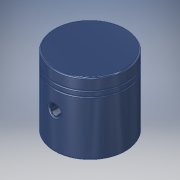
# Autodesk Inventor part: Se-Elmer-Radical-Engine:Piston
Saved by Autodesk Inventor 2017 (Build 210142000, 142)
## iProperties
Created: 2020-01-12
Material: Stainless Steel
Document SubType Name: Modeling
Designer: Admin
Density: 8 g/cm^3
Appearance: Flaked Satin - Blue
Mass: 15.0776 g
Surface Area: 16.4031 cm^2
Volume: 1.88469 cm^3
Author: Admin
Autodesk Inventor part; units mm, degrees
ref_plane "YZ Plane" through (0, 0, 0) normal (1, 0, 0) x (0, 1, 0)
sketch "Sketch1" plane through (0, 0, 0) normal (0, 1, 0) x (-1, 0, 0)
  circle A0 centre (0, 0) radius 7.9375
  dimension "d0" = 15.875
  constraints: 1 centre point, 1 coincident
  measures "d0" diameter of A0
extrude "Extrusion1" add sketch "Sketch1" along normal mid plane 15.875
sketch "Sketch2" plane through (0, -7.9375, 0) normal (0, -1, 0) x (1, 0, 0)
  point P0 (0, 0)
  point P1 (0, 0)
  constraints: 1 coincident
hole "Hole1" at (0, -7.9375, 0) direction (0, 1, 0) diameter 9.525 depth 13.4938 counterbore diameter 12.7 counterbore depth 4.7625
ref_plane "Work Plane1" through (0, 0, -7.9375) normal (0, 0, 1) x (1, 0, 0)
sketch "Sketch3" plane through (0, 0, -7.9375) normal (0, 0, 1) x (1, 0, 0)
  point P0 (0, 0)
  point P1 (0, 0)
  dimension "d11" = 0
  dimension "d12" = 0
  measures "d11" distance of point (0, 0) point (0, 0)
  measures "d12" distance of point (0, 0) point (0, 0)
hole "Hole2" at (0, 0, -7.9375) direction (0, 0, 1) diameter 2.3813 end through all
sketch "Sketch4" plane through (0, 0, 0) normal (1, 0, 0) x (0, 1, 0)
  line L0 (5.5562, 7.9375) -> (5.3657, 7.747)
  line L1 (5.3657, 7.747) -> (5.1753, 7.9375)
  line L2 (5.1753, 7.9375) -> (5.5562, 7.9375)
  line L3 (4.7784, 15.0093) -> (4.7784, -11.52)
  line L4 (4.0005, 7.9375) -> (4.191, 7.747)
  line L5 (4.191, 7.747) -> (4.3815, 7.9375)
  line L6 (4.3815, 7.9375) -> (4.0005, 7.9375)
  line L7 (-11.1125, 0) -> (11.1125, 0) projected
  point P0 (0, 0)
  dimension "d20" = 0.381
  dimension "d21" = 0.1905
  dimension "d22" = 7.9375
  dimension "d23" = 5.5563
  dimension "d24" = 0.3969
  constraints: 14 end point, 3 symmetric about line, 1 horizontal, 1 perpendicular, 1 vertical
  measures "d20" distance of L1.end L0.start
  measures "d21" distance from line of L0.end L2
  measures "d22" distance from line of point (0, 0) L2
  measures "d23" horizontal distance of point (0, 0) L0.start
  measures "d24" distance from line of L1.end L3
revolve "Revolution1" cut sketch "Sketch4" angle 360 about axis through (0, -10, 0) along (0, 1, 0)
ref_plane "Work Plane2" through (0, 0, -7.9375) normal (0, 0, 1) x (1, 0, 0)
fillet "Fillet1" radius 0.3175 17 edges at (7.9375, 7.9375, 0) (7.9375, -7.9375, 0) (0, 5.3657, -7.747) (0, 4.191, -7.747) (0, -3.175, 6.35) (0, -3.175, 4.7625) (0, 5.5563, 4.7625) (-0.8908, 0.79, 7.8874) (0.8908, 0.7899, 7.8874) (0, -1.1906, 7.9375) (0.8908, 0.7899, -7.8874) (0.8908, -0.79, -7.8874) (-0.8908, 0.79, -7.8874) (-0.8908, -0.79, -7.8874) (-0.0006, -1.1906, 4.7625) (-1.1906, 0.0001, -4.6113) (1.1906, 0.0001, -4.6113)
fillet_without_effect "Fillet2"
body "Solid1"
